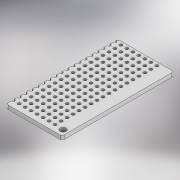
# Autodesk Inventor part: Modulo NRF24 2
Saved by Autodesk Inventor 2021.4 (Build 254397000, 397)
## iProperties
Created: 2022-11-18
Part Number: Modulo NRF24 2
Material: Genérico
Document SubType Name: Modeling
Designer: crist
Density: 1 g/cm^3
Appearance: Valor por defecto
Author: crist
Autodesk Inventor part; units mm, degrees
ref_plane "YZ Plane" through (0, 0, 0) normal (1, 0, 0) x (0, 1, 0)
ref_plane "XZ Plane" through (0, 0, 0) normal (0, 1, 0) x (-1, 0, 0)
ref_plane "XY Plane" through (0, 0, 0) normal (0, 0, 1) x (1, 0, 0)
sketch "Boceto1" plane through (0, 0, 0) normal (0, 1, 0) x (-1, 0, 0)
  line L0 (1, 0) -> (27, 0)
  line L1 (28, -1) -> (28, -55)
  line L2 (27, -56) -> (1, -56)
  line L3 (0, -55) -> (0, -1)
  arc A0 (28, -1) -> (27, 0) centre (27, -1) ccw
  arc A1 (27, -56) -> (28, -55) centre (27, -55) ccw
  arc A2 (0, -55) -> (1, -56) centre (1, -55) ccw
  arc A3 (1, 0) -> (0, -1) centre (1, -1) ccw
  line L4 (0, 0) -> (0, -1.5)
  line L5 (0, -1.5) -> (0, -3)
  line L6 (0, -3) -> (2.5, -3)
  circle A4 centre (2.5, -3) radius 1.5
  point P0 (28, -56)
  point P1 (28, 0)
  point P2 (0, -56)
  dimension "d0" = 56
  dimension "d1" = 28
  dimension "d2" = 1
  dimension "d19" = 1.5
  dimension "d20" = 1.5
  dimension "d21" = 2.5
  dimension "d22" = 3
  constraints: 14 end point, 10 point on line, 8 point on circle, 8 tangent, 5 centre point, 3 equal radius, 2 parallel, 2 perpendicular, 1 coincident, 1 horizontal
  measures "d0" distance of point (28, 0) point (28, -56)
  measures "d1" distance of point (28, -56) point (0, -56)
  measures "d2" radius of A0
  measures "d19" distance of L4.start L4.end
  measures "d20" distance of L4.end L5.end
  measures "d21" distance of L5.end L6.end
  measures "d22" diameter of A4
extrude "Extrusión1" add sketch "Boceto1" along normal blind 2
sketch "Boceto3" plane through (0, 2, 0) normal (0, 1, 0) x (1, 0, 0)
  line L0 (0, 0) -> (-6.75, 0)
  line L1 (-27, 0) -> (-1, 0) projected
  line L2 (-6.75, 0) -> (-6.75, 3.25)
  circle A0 centre (-6.75, 3.25) radius 0.75
  line L3 (0, 0) -> (0, 4.634)
  line L4 (0, 1) -> (0, 55) projected
  circle A1 centre (-9.75, 3.25) radius 0.75
  circle A2 centre (-12.75, 3.25) radius 0.75
  circle A3 centre (-15.75, 3.25) radius 0.75
  circle A4 centre (-18.75, 3.25) radius 0.75
  circle A5 centre (-21.75, 3.25) radius 0.75
  circle A6 centre (-24.75, 3.25) radius 0.75
  circle A7 centre (-27.75, 3.25) radius 0.75
  circle A8 centre (-6.75, 6.25) radius 0.75
  circle A9 centre (-9.75, 6.25) radius 0.75
  circle A10 centre (-12.75, 6.25) radius 0.75
  circle A11 centre (-15.75, 6.25) radius 0.75
  circle A12 centre (-18.75, 6.25) radius 0.75
  circle A13 centre (-21.75, 6.25) radius 0.75
  circle A14 centre (-24.75, 6.25) radius 0.75
  circle A15 centre (-27.75, 6.25) radius 0.75
  circle A16 centre (-6.75, 9.25) radius 0.75
  circle A17 centre (-9.75, 9.25) radius 0.75
  circle A18 centre (-12.75, 9.25) radius 0.75
  circle A19 centre (-15.75, 9.25) radius 0.75
  circle A20 centre (-18.75, 9.25) radius 0.75
  circle A21 centre (-21.75, 9.25) radius 0.75
  circle A22 centre (-24.75, 9.25) radius 0.75
  circle A23 centre (-27.75, 9.25) radius 0.75
  circle A24 centre (-6.75, 12.25) radius 0.75
  circle A25 centre (-9.75, 12.25) radius 0.75
  circle A26 centre (-12.75, 12.25) radius 0.75
  circle A27 centre (-15.75, 12.25) radius 0.75
  circle A28 centre (-18.75, 12.25) radius 0.75
  circle A29 centre (-21.75, 12.25) radius 0.75
  circle A30 centre (-24.75, 12.25) radius 0.75
  circle A31 centre (-27.75, 12.25) radius 0.75
  circle A32 centre (-6.75, 15.25) radius 0.75
  circle A33 centre (-9.75, 15.25) radius 0.75
  circle A34 centre (-12.75, 15.25) radius 0.75
  circle A35 centre (-15.75, 15.25) radius 0.75
  circle A36 centre (-18.75, 15.25) radius 0.75
  circle A37 centre (-21.75, 15.25) radius 0.75
  circle A38 centre (-24.75, 15.25) radius 0.75
  circle A39 centre (-27.75, 15.25) radius 0.75
  circle A40 centre (-6.75, 18.25) radius 0.75
  circle A41 centre (-9.75, 18.25) radius 0.75
  circle A42 centre (-12.75, 18.25) radius 0.75
  circle A43 centre (-15.75, 18.25) radius 0.75
  circle A44 centre (-18.75, 18.25) radius 0.75
  circle A45 centre (-21.75, 18.25) radius 0.75
  circle A46 centre (-24.75, 18.25) radius 0.75
  circle A47 centre (-27.75, 18.25) radius 0.75
  circle A48 centre (-6.75, 21.25) radius 0.75
  circle A49 centre (-9.75, 21.25) radius 0.75
  circle A50 centre (-12.75, 21.25) radius 0.75
  circle A51 centre (-15.75, 21.25) radius 0.75
  circle A52 centre (-18.75, 21.25) radius 0.75
  circle A53 centre (-21.75, 21.25) radius 0.75
  circle A54 centre (-24.75, 21.25) radius 0.75
  circle A55 centre (-27.75, 21.25) radius 0.75
  circle A56 centre (-6.75, 24.25) radius 0.75
  circle A57 centre (-9.75, 24.25) radius 0.75
  circle A58 centre (-12.75, 24.25) radius 0.75
  circle A59 centre (-15.75, 24.25) radius 0.75
  circle A60 centre (-18.75, 24.25) radius 0.75
  circle A61 centre (-21.75, 24.25) radius 0.75
  circle A62 centre (-24.75, 24.25) radius 0.75
  circle A63 centre (-27.75, 24.25) radius 0.75
  circle A64 centre (-6.75, 27.25) radius 0.75
  circle A65 centre (-9.75, 27.25) radius 0.75
  circle A66 centre (-12.75, 27.25) radius 0.75
  circle A67 centre (-15.75, 27.25) radius 0.75
  circle A68 centre (-18.75, 27.25) radius 0.75
  circle A69 centre (-21.75, 27.25) radius 0.75
  circle A70 centre (-24.75, 27.25) radius 0.75
  circle A71 centre (-27.75, 27.25) radius 0.75
  circle A72 centre (-6.75, 30.25) radius 0.75
  circle A73 centre (-9.75, 30.25) radius 0.75
  circle A74 centre (-12.75, 30.25) radius 0.75
  circle A75 centre (-15.75, 30.25) radius 0.75
  circle A76 centre (-18.75, 30.25) radius 0.75
  circle A77 centre (-21.75, 30.25) radius 0.75
  circle A78 centre (-24.75, 30.25) radius 0.75
  circle A79 centre (-27.75, 30.25) radius 0.75
  circle A80 centre (-6.75, 33.25) radius 0.75
  circle A81 centre (-9.75, 33.25) radius 0.75
  circle A82 centre (-12.75, 33.25) radius 0.75
  circle A83 centre (-15.75, 33.25) radius 0.75
  circle A84 centre (-18.75, 33.25) radius 0.75
  circle A85 centre (-21.75, 33.25) radius 0.75
  circle A86 centre (-24.75, 33.25) radius 0.75
  circle A87 centre (-27.75, 33.25) radius 0.75
  circle A88 centre (-6.75, 36.25) radius 0.75
  circle A89 centre (-9.75, 36.25) radius 0.75
  circle A90 centre (-12.75, 36.25) radius 0.75
  circle A91 centre (-15.75, 36.25) radius 0.75
  circle A92 centre (-18.75, 36.25) radius 0.75
  circle A93 centre (-21.75, 36.25) radius 0.75
  circle A94 centre (-24.75, 36.25) radius 0.75
  circle A95 centre (-27.75, 36.25) radius 0.75
  circle A96 centre (-6.75, 39.25) radius 0.75
  circle A97 centre (-9.75, 39.25) radius 0.75
  circle A98 centre (-12.75, 39.25) radius 0.75
  circle A99 centre (-15.75, 39.25) radius 0.75
  circle A100 centre (-18.75, 39.25) radius 0.75
  circle A101 centre (-21.75, 39.25) radius 0.75
  circle A102 centre (-24.75, 39.25) radius 0.75
  circle A103 centre (-27.75, 39.25) radius 0.75
  circle A104 centre (-6.75, 42.25) radius 0.75
  circle A105 centre (-9.75, 42.25) radius 0.75
  circle A106 centre (-12.75, 42.25) radius 0.75
  circle A107 centre (-15.75, 42.25) radius 0.75
  circle A108 centre (-18.75, 42.25) radius 0.75
  circle A109 centre (-21.75, 42.25) radius 0.75
  circle A110 centre (-24.75, 42.25) radius 0.75
  circle A111 centre (-27.75, 42.25) radius 0.75
  circle A112 centre (-6.75, 45.25) radius 0.75
  circle A113 centre (-9.75, 45.25) radius 0.75
  circle A114 centre (-12.75, 45.25) radius 0.75
  circle A115 centre (-15.75, 45.25) radius 0.75
  circle A116 centre (-18.75, 45.25) radius 0.75
  circle A117 centre (-21.75, 45.25) radius 0.75
  circle A118 centre (-24.75, 45.25) radius 0.75
  circle A119 centre (-27.75, 45.25) radius 0.75
  circle A120 centre (-6.75, 48.25) radius 0.75
  circle A121 centre (-9.75, 48.25) radius 0.75
  circle A122 centre (-12.75, 48.25) radius 0.75
  circle A123 centre (-15.75, 48.25) radius 0.75
  circle A124 centre (-18.75, 48.25) radius 0.75
  circle A125 centre (-21.75, 48.25) radius 0.75
  circle A126 centre (-24.75, 48.25) radius 0.75
  circle A127 centre (-27.75, 48.25) radius 0.75
  circle A128 centre (-6.75, 51.25) radius 0.75
  circle A129 centre (-9.75, 51.25) radius 0.75
  circle A130 centre (-12.75, 51.25) radius 0.75
  circle A131 centre (-15.75, 51.25) radius 0.75
  circle A132 centre (-18.75, 51.25) radius 0.75
  circle A133 centre (-21.75, 51.25) radius 0.75
  circle A134 centre (-24.75, 51.25) radius 0.75
  circle A135 centre (-27.75, 51.25) radius 0.75
  circle A136 centre (-6.75, 54.25) radius 0.75
  circle A137 centre (-9.75, 54.25) radius 0.75
  circle A138 centre (-12.75, 54.25) radius 0.75
  circle A139 centre (-15.75, 54.25) radius 0.75
  circle A140 centre (-18.75, 54.25) radius 0.75
  circle A141 centre (-21.75, 54.25) radius 0.75
  circle A142 centre (-24.75, 54.25) radius 0.75
  circle A143 centre (-27.75, 54.25) radius 0.75
  dimension "d32" = 6.75
  dimension "d33" = 3.25
  dimension "d34" = 1.5
  dimension "d37" = 3
  dimension "d40" = 3
  constraints: 144 centre point, 6 end point, 2 point on line, 1 coincident, 1 horizontal, 1 perpendicular, 1 vertical, 286 other
  measures "d32" distance of L0.start L0.end
  measures "d33" distance of L0.end L2.end
  measures "d34" diameter of A0
  measures "d37" distance of A0.centre A1.centre
  measures "d40" distance of A0.centre A8.centre
extrude "Extrusión3" cut sketch "Boceto3" against normal blind 2
